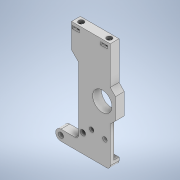
# Autodesk Inventor part: PartB
Saved by Autodesk Inventor 2020.2 (Build 242310000, 310)
## iProperties
Created: 2020-12-02
Part Number: PartB
Material: Generic
Document SubType Name: Modeling
Designer: Acer
Density: 1 g/cm^3
Appearance: Default
Author: Acer
Autodesk Inventor part; units mm, degrees
ref_plane "YZ Plane" through (0, 0, 0) normal (1, 0, 0) x (0, 1, 0)
ref_plane "XZ Plane" through (0, 0, 0) normal (0, 1, 0) x (-1, 0, 0)
ref_plane "XY Plane" through (0, 0, 0) normal (0, 0, 1) x (1, 0, 0)
sketch "Sketch1" plane through (0, 0, 0) normal (0, 0, 1) x (1, 0, 0)
  circle A0 centre (0, 0) radius 1.5
  circle A1 centre (0, 0) radius 3
  line L0 (0, 3) -> (28, 3)
  line L1 (28, 3) -> (28, -3)
  line L2 (28, -3) -> (0, -3)
  line L3 (0, -3) -> (0, 3)
  line L4 (28, 3) -> (10, 3)
  line L5 (10, 3) -> (10, 59)
  line L6 (10, 59) -> (28, 59)
  line L7 (28, 59) -> (28, 3)
  circle A2 centre (23.5, 28.5) radius 5.5
  circle A3 centre (18.553, 47) radius 6.25
  line L8 (23.5, 28.5) -> (18.553, 47) construction
  line L9 (23.5, 28.5) -> (10, 28.5) construction
  circle A4 centre (10.053, 47) radius 1
  circle A5 centre (22.803, 39.6388) radius 1
  circle A6 centre (22.803, 54.3612) radius 1
  line L10 (10, 59) -> (6, 59)
  line L11 (6, 59) -> (6, 45)
  line L12 (6, 45) -> (10, 45)
  line L13 (10, 45) -> (10, 59)
  line L14 (6, 45) -> (10, 41)
  line L15 (6, 45) -> (11.6569, 45) construction
  line L16 (28, 34.5) -> (31, 34.5)
  line L17 (31, 34.5) -> (31, 22.5)
  line L18 (31, 22.5) -> (28, 22.5)
  line L19 (28, 22.5) -> (28, 34.5)
  line L20 (31, 34.5) -> (28, 37.5)
  line L21 (31, 34.5) -> (35.2426, 34.5) construction
  line L22 (31, 22.5) -> (28, 19.5)
  line L23 (31, 22.5) -> (35.2426, 22.5) construction
  circle A7 centre (12.5, 7.5) radius 1.5
  circle A8 centre (17.5, 11.5) radius 1.25
  circle A9 centre (25, 10.5) radius 1.25
  line L24 (18.553, 47) -> (6, 47) construction
  line L25 (10.053, 47) -> (18.553, 47) construction
  dimension "d0" = 3
  dimension "d1" = 6
  dimension "d2" = 28
  dimension "d3" = 6
  dimension "d4" = 0
  dimension "d5" = 3
  dimension "d6" = 18
  dimension "d7" = 56
  dimension "d8" = 11
  dimension "d9" = 4.5
  dimension "d10" = 25.5
  dimension "d11" = 12.5
  dimension "d12" = 19.15
  dimension "d14" = 2
  dimension "d17" = 12
  dimension "d20" = 360
  dimension "d22" = 4
  dimension "d23" = 14
  dimension "d24" = 45
  dimension "d25" = 3
  dimension "d26" = 12
  dimension "d27" = 6
  dimension "d28" = 135
  dimension "d29" = 135
  dimension "d32" = 3
  dimension "d33" = 10.5
  dimension "d34" = 2.5
  dimension "d35" = 2.5
  dimension "d36" = 14.5
  dimension "d37" = 7.5
  dimension "d38" = 2.5
  dimension "d39" = 15
  dimension "d40" = 13.5
  dimension "d60" = 8.5
  dimension "d61" = 0
  constraints: 52 end point, 10 centre point, 8 horizontal, 8 parallel, 6 point on line, 5 perpendicular, 3 equal length, 2 coincident, 7 other
  measures "d0" diameter of A0
  measures "d1" diameter of A1
  measures "d2" distance of L1.end L2.end
  measures "d3" distance of L0.end L1.end
  measures "d4" distance from line of point (0, 0) L3
  measures "d5" distance from line of L0 point (0, 0)
  measures "d6" distance of L5.end L6.end
  measures "d7" distance of L4.end L5.end
  measures "d8" diameter of A2
  measures "d9" distance from line of L7 L8.start
  measures "d10" distance from line of L8.start L0
  measures "d11" diameter of A3
  measures "d12" distance of L8.start L8.end
  measures "d14" diameter of A4
  measures "d17" distance from line of L6 L8.end
  measures "d22" distance of L12.end L11.end
  measures "d23" distance of L11.end L10.end
  measures "d24" angle of L14 L15
  measures "d25" distance of L17.end L18.end
  measures "d26" distance of L16.end L17.end
  measures "d27" distance from line of L16 L8.start
  measures "d28" angle of L21 L20
  measures "d29" angle of L22 L23
  measures "d32" diameter of A7
  measures "d33" distance from line of L2 A7.centre
  measures "d34" distance from line of L5 A7.centre
  measures "d35" diameter of A8
  measures "d36" distance from line of A8.centre L2
  measures "d37" distance from line of L5 A8.centre
  measures "d38" diameter of A9
  measures "d39" distance from line of A9.centre L5
  measures "d40" distance from line of L2 A9.centre
  measures "d60" distance of L25.start L8.end
  measures "d61" distance between parallel lines of L24 L25
extrude "Extrusion1" add sketch "Sketch1" along normal blind 5 contours A0 L3 A1 | A0 L3 A1 | L0 L1 L2 A1 | L5 A4 L6 L7 A2 L0 | L14 L12 L5 | L7 L18 L22 | L12 L11 L10 L5 A4 | L7 A2 L16 L17 L18 | A4 L5 | L5 A4 | L16 L7 L20 | A3 | A5 | A6
fillet "Fillet1" radius 2 1 edges at (28, -3, 2.5)
fillet "Fillet2" radius 2 1 edges at (10, 3, 2.5)
sketch "Sketch2" plane through (0, 0, 5) normal (0, 0, 1) x (1, 0, 0)
  line L0 (28, -1) -> (28, 19.5) projected
  line L1 (0, -3) -> (26, -3) projected
  line L2 (28, -1) -> (28, 19.5) projected
  line L3 (28, 20.75) -> (15.25, 20.75)
  line L4 (15.25, 20.75) -> (15.25, 0.75)
  line L5 (15.25, 0.75) -> (28, 0.75)
  line L6 (28, 0.75) -> (28, 20.75)
  line L7 (28, 19.5) -> (31, 22.5) projected
  line L8 (28, 20.75) -> (29.25, 20.75)
  line L9 (28, 19.5) -> (31, 22.5) projected
  point P0 (0, 0)
  dimension "d43" = 12.75
  dimension "d44" = 20
  dimension "d45" = 23.75
  constraints: 10 end point, 2 horizontal, 2 parallel, 2 point on line, 1 perpendicular
  measures "d43" distance of L5.end L4.end
  measures "d44" distance of L4.end L3.end
  measures "d45" distance between parallel lines of L1 L3
extrude "Extrusion2" cut sketch "Sketch2" against normal blind 3
sketch "Sketch3" plane through (6, 59, 0) normal (0, 1, 0) x (1, 0, 0)
  circle A0 centre (3, -2.5) radius 1.5
  line L0 (22, 0) -> (0, 0) projected
  line L1 (0, 0) -> (0, -5) projected
  line L2 (22, -5) -> (0, -5) projected
  line L3 (22, 0) -> (22, -5) projected
  circle A1 centre (19, -2.5) radius 1.5
  dimension "d48" = 3
  dimension "d49" = 3
  dimension "d50" = 2.5
  dimension "d51" = 2.5
  dimension "d52" = 3
  dimension "d53" = 3
  constraints: 2 centre point
  measures "d48" diameter of A0
  measures "d49" diameter of A1
  measures "d50" distance from line of L0 A0.centre
  measures "d51" distance from line of L0 A1.centre
  measures "d52" distance from line of A1.centre L3
  measures "d53" distance from line of L1 A0.centre
extrude "Extrusion3" cut sketch "Sketch3" against normal blind 4 contours A0 | A1
thread "Thread1" size "M3x0.5" class "6H" standard "ANSI Metric M Profile" length 7
thread "Thread2" size "M3x0.5" class "6H" standard "ANSI Metric M Profile" length 7
mirror "Mirror1" about plane through (14, 28, 0) normal (0, 0, -1) remove original yes
sketch "Sketch5" plane through (26, -3, -5) normal (0, 0, -1) x (-1, 0, 0)
  line L0 (2.5, 58) -> (2.5, 62) projected
  line L1 (-0.5, 58) -> (-0.5, 62) projected
  line L2 (15.5, 58) -> (15.5, 62) projected
  line L3 (18.5, 58) -> (18.5, 62) projected
  line L4 (-0.5, 60.3) -> (3.5, 60.3)
  line L5 (3.5, 60.3) -> (3.5, 58.7)
  line L6 (3.5, 58.7) -> (-0.5, 58.7)
  line L7 (-0.5, 58.7) -> (-0.5, 60.3)
  line L8 (-0.5, 60.3) -> (3.5, 58.7) construction
  line L9 (3.5, 60.3) -> (-0.5, 58.7) construction
  line L10 (15.5, 60.3) -> (19.5, 60.3)
  line L11 (19.5, 60.3) -> (19.5, 58.7)
  line L12 (19.5, 58.7) -> (15.5, 58.7)
  line L13 (15.5, 58.7) -> (15.5, 60.3)
  line L14 (15.5, 60.3) -> (19.5, 58.7) construction
  line L15 (19.5, 60.3) -> (15.5, 58.7) construction
  line L16 (-2, 62) -> (20, 62) projected
  point P0 (26, 3)
  point P1 (1.5, 59.5)
  point P2 (17.5, 59.5)
  dimension "d62" = 4
  dimension "d63" = 1.6
  dimension "d64" = 4
  dimension "d65" = 1.6
  dimension "d66" = 1
  dimension "d67" = 1.7
  dimension "d68" = 1
  dimension "d69" = 1.7
  constraints: 24 end point, 4 midpoint, 4 parallel, 2 horizontal, 2 perpendicular
  measures "d62" distance of L5.end L6.end
  measures "d63" distance of L4.end L5.end
  measures "d64" distance of L11.end L12.end
  measures "d65" distance of L10.end L11.end
  measures "d66" distance from line of L0 point (1.5, 59.5)
  measures "d67" distance between parallel lines of L16 L4
  measures "d68" distance from line of point (17.5, 59.5) L3
  measures "d69" distance between parallel lines of L16 L10
extrude "Extrusion4" cut sketch "Sketch5" against normal up to surface (5 mm away) contours L6 L1 L4 L0 | L0 L4 L5 L6 | L2 L10 L3 L12 | L3 L10 L11 L12
sketch "Sketch6" plane through (26, -3, -5) normal (0, 0, -1) x (-1, 0, 0)
  circle A0 centre (13.5, 10.5) radius 1.5 projected
  circle A1 centre (13.5, 10.5) radius 2.75
  point P0 (26, 3)
  dimension "d72" = 5.5
  constraints: 1 centre point, 1 coincident
  measures "d72" diameter of A1
extrude "Extrusion5" cut sketch "Sketch6" against normal blind 2 contours A0 | A1
body "Solid1"
